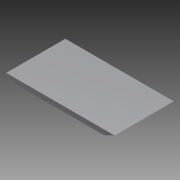
# Autodesk Inventor part: Bridge
Saved by Autodesk Inventor 2012 (Build 160160000, 160)
## iProperties
Created: 2012-01-07
Part Number: Bridge
Material: Default
Document SubType Name: Modeling
Designer: Justin
Density: 1 g/cm^3
Author: Justin
Autodesk Inventor part; units mm, degrees
ref_plane "YZ Plane" through (0, 0, 0) normal (1, 0, 0) x (0, 1, 0)
ref_plane "XZ Plane" through (0, 0, 0) normal (0, 1, 0) x (-1, 0, 0)
ref_plane "XY Plane" through (0, 0, 0) normal (0, 0, 1) x (1, 0, 0)
sketch "Sketch1" plane through (0, 0, 0) normal (0, 0, 1) x (1, 0, 0)
  line L0 (0, 0) -> (2235.2, 0)
  line L1 (0, 0) -> (218.4618, -102.4702)
  line L2 (2235.2, 0) -> (2016.7382, -102.4702)
  line L3 (218.4618, -102.4702) -> (2016.7382, -102.4702)
  line L4 (1016.751, -102.4702) -> (1016.751, -305.6702)
  line L5 (1016.751, -305.6702) -> (1067.551, -305.6702)
  line L6 (1067.551, -305.6702) -> (1067.551, -102.4702)
  dimension "d1" = 2235.2
  dimension "d2" = 241.3
  dimension "d3" = 241.3
  dimension "d7" = 203.2
  dimension "d8" = 50.8
  constraints: 14 end point, 3 perpendicular, 2 point on line, 1 horizontal, 1 parallel
  measures "d1" distance of L0.start L0.end
  measures "d2" distance of L0.start L1.end
  measures "d3" distance of L0.end L2.end
  measures "d7" distance of L4.start L4.end
  measures "d8" distance of L4.end L5.end
extrude "Extrusion1" add sketch "Sketch1" along normal blind 1219.2 contours L0 L2 L3 L1
body "Solid1"
